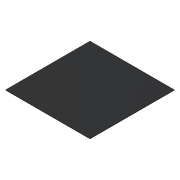
# Autodesk Inventor part: M10 - Base Rubber
Saved by Autodesk Inventor 2016 (Build 200138000, 138)
## iProperties
Created: 2016-12-26
Part Number: M10 - Base Rubber
Material: Rubber
Document SubType Name: Modeling
Designer: Fernando
Stock Number: 0
Mass: 82.026 g
Surface Area: 898.8 cm^2
Volume: 88.2 cm^3
Density: 0.93 g/cm^3
Appearance: Rubber - Black
SurfaceArea_m2: .09
Author: Fernando
Autodesk Inventor part; units mm, degrees
ref_plane "YZ Plane" through (0, 0, 0) normal (1, 0, 0) x (0, 1, 0)
ref_plane "XZ Plane" through (0, 0, 0) normal (0, 1, 0) x (-1, 0, 0)
ref_plane "XY Plane" through (0, 0, 0) normal (0, 0, 1) x (1, 0, 0)
sketch "Sketch2" plane through (0, 0, 0) normal (0, 0, 1) x (1, 0, 0)
  line L0 (-105, 105) -> (105, 105)
  line L1 (105, 105) -> (105, -105)
  line L2 (105, -105) -> (-105, -105)
  line L3 (-105, -105) -> (-105, 105)
  line L4 (-105, 105) -> (105, -105) construction
  line L5 (105, 105) -> (-105, -105) construction
  point P0 (0, 0)
  dimension "d11" = 210
  constraints: 12 end point, 2 midpoint, 2 parallel, 2 perpendicular, 1 horizontal
  measures "d11" distance of L0.start L0.end
extrude "Extrusion2" add sketch "Sketch2" along normal blind 2
body "Solid2"
